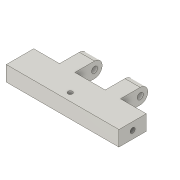
# Autodesk Inventor part: Führungsbock
Saved by Autodesk Inventor 2018.3 (Build 223284000, 284)
## iProperties
Created: 2019-11-28
Material: Stahl, unlegiert
Document SubType Name: Modeling
Designer: dirkb
Density: 7.85 g/cm^3
Appearance: Stahl
Description: Führungsbock
Werkstoff: S235JRC+C
Author: dirkb
Autodesk Inventor part; units mm, degrees
ref_plane "YZ Plane" through (0, 0, 0) normal (1, 0, 0) x (0, 1, 0)
ref_plane "XZ Plane" through (0, 0, 0) normal (0, 1, 0) x (-1, 0, 0)
ref_plane "XY Plane" through (0, 0, 0) normal (0, 0, 1) x (1, 0, 0)
sketch "Skizze_Grundkörper" plane through (0, 0, 0) normal (0, 0, 1) x (1, 0, 0)
  line L0 (-51.8, 0) -> (51.8, 0) projected
  line L1 (0, -25.2) -> (0, 25.2) projected
  line L2 (37, -18) -> (-37, -18)
  line L3 (-37, -18) -> (-37, 18)
  line L4 (-37, 18) -> (37, 18)
  line L5 (37, 18) -> (37, -18)
  line L6 (37, -18) -> (-37, 18) construction
  line L7 (-37, -18) -> (37, 18) construction
  point P0 (0, 0)
  dimension "Länge" = 74
  dimension "Höhe" = 36
  constraints: 12 end point, 2 midpoint, 2 parallel, 1 horizontal, 1 perpendicular
  measures "Länge" distance of L3.end L4.end
  measures "Höhe" distance of L4.end L2.start
extrude "Grundkörper" add sketch "Skizze_Grundkörper" along normal mid plane 10
sketch "Skizze_Ausnehmung" plane through (0, 0, 5) normal (0, 0, 1) x (1, 0, 0)
  line L0 (-51.8, 0) -> (51.8, 0) projected
  line L1 (0, -25.2) -> (0, 25.2) projected
  line L2 (-37, -18) -> (37, -18) projected
  line L3 (37, -18) -> (37, 18) projected
  line L4 (37, 18) -> (-37, 18) projected
  line L5 (-37, 18) -> (-37, -18) projected
  line L6 (10, 0) -> (-10, 0)
  line L7 (-10, 0) -> (-10, 18)
  line L8 (-10, 18) -> (10, 18)
  line L9 (10, 18) -> (10, 0)
  line L10 (10, 0) -> (-10, 18) construction
  line L11 (-10, 0) -> (10, 18) construction
  line L12 (-37, 18) -> (-20, 18)
  line L13 (-20, 18) -> (-20, 0)
  line L14 (-20, 0) -> (-37, 0)
  line L15 (-37, 0) -> (-37, 18)
  line L16 (37, 18) -> (20, 18)
  line L17 (20, 18) -> (20, 0)
  line L18 (20, 0) -> (37, 0)
  line L19 (37, 0) -> (37, 18)
  point P0 (0, 0)
  point P1 (0, 9)
  dimension "d4" = 18
  dimension "d5" = 20
  dimension "d6" = 40
  constraints: 28 end point, 6 parallel, 3 horizontal, 3 perpendicular, 3 point on line, 2 midpoint, 1 collinear, 1 other
  measures "d4" distance between parallel lines of L2 L6
  measures "d5" distance between parallel lines of L9 L7
  measures "d6" distance between parallel lines of L17 L13
extrude "Ausnehmung" cut sketch "Skizze_Ausnehmung" against normal through all contours L5 L4 L13 L0 | L7 L4 L1 L0 | L1 L4 L9 L0 | L0 L17 L4 L3
full round fillet "Rundung1" first side at (-3.3333, -12, 5) centre faces at (-13.3333, 18, 1.6667) second side at (-3.3333, -12, -5)
full round fillet "Rundung2" first side at (-3.3333, -12, 5) centre faces at (13.3333, 18, -1.6667) second side at (-3.3333, -12, -5)
hole "Bohrung_4_mm" at (20, 13, 0) direction (-1, 0, 0) diameter 4 end through all
sketch "Skizze_Bohrung_3_mm" plane through (0, 0, 5) normal (0, 0, 1) x (1, 0, 0)
  line L0 (10, 13) -> (20, 13) projected
  line L1 (10, 13) -> (10, 0) projected
  line L2 (10, 0) -> (-10, 0) projected
  line L3 (-10, 0) -> (-10, 13) projected
  line L4 (-20, 13) -> (-10, 13) projected
  line L5 (-20, 13) -> (-20, 0) projected
  line L6 (-20, 0) -> (-37, 0) projected
  line L7 (-37, 0) -> (-37, -18) projected
  line L8 (-37, -18) -> (37, -18) projected
  line L9 (37, -18) -> (37, 0) projected
  line L10 (37, 0) -> (20, 0) projected
  line L11 (20, 0) -> (20, 13) projected
  line L12 (-51.8, 0) -> (51.8, 0) projected
  line L13 (0, -25.2) -> (0, 25.2) projected
  point P0 (0, 0)
  point P1 (0, -13)
  dimension "d18" = 5
  constraints: 1 point on line, 1 other
  measures "d18" distance from line of point (0, -13) L8
hole "Bohrung_3_mm" at (0, -13, 5) direction (0, 0, -1) diameter 3 end through all
sketch "Skizze4" plane through (37, -18, 5) normal (1, 0, 0) x (0, 0, -1)
  line L0 (5, -7.2) -> (5, 43.2) projected
  line L1 (12, 18) -> (-2, 18) projected
  line L2 (10, 18) -> (0, 18) projected
  line L3 (0, 0) -> (0, 18) projected
  line L4 (10, 0) -> (0, 0) projected
  line L5 (10, 18) -> (10, 0) projected
  point P0 (5, 18)
  point P1 (5, 9)
  dimension "d26" = 9
  constraints: 1 point on line
  measures "d26" distance from line of L4 point (5, 9)
hole "Bohrung_M4" at (37, -9, 0) direction (-1, 0, 0) diameter 3.242 depth 14 tip angle 118 thread size "M4x0.7" class "6H" standard "ISO Metric profile"
pattern_circular "Runde Anordnung_M4" count 2 over 360 about axis through (0, -10, 0) along (0, 1, 0) of "Bohrung_M4"
